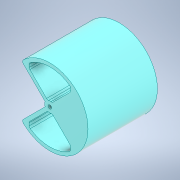
# Autodesk Inventor part: Feeder Rotator
Saved by Autodesk Inventor 2020.3 (Build 243373000, 373)
## iProperties
Created: 2020-07-23
Part Number: Feeder Rotator
Material: ABS Plastic
Document SubType Name: Modeling
Designer: juanp
Density: 1.06 g/cm^3
Appearance: Smooth - White
Author: juanp
Autodesk Inventor part; units mm, degrees
ref_plane "YZ Plane" through (0, 0, 0) normal (1, 0, 0) x (0, 1, 0)
ref_plane "XZ Plane" through (0, 0, 0) normal (0, 1, 0) x (-1, 0, 0)
ref_plane "XY Plane" through (0, 0, 0) normal (0, 0, 1) x (1, 0, 0)
sketch "Sketch2" plane through (0, 0, 0) normal (0, 0, 1) x (1, 0, 0)
  arc A0 (20.126, -22.2473) -> (-20.126, -22.2473) centre (0, 0) ccw construction
  arc A1 (-24.3711, -22.2497) -> (-24.3711, 22.2497) centre (0, 0) ccw
  line L0 (32.9543, 32.9543) -> (23.3345, 23.3345) construction
  line L1 (-32.8174, 32.8174) -> (-23.3345, 23.3345) construction
  line L2 (23.3345, 23.3345) -> (-23.3345, -23.3345) construction
  line L3 (23.3345, -23.3345) -> (30.6779, -35.5804) construction
  line L4 (-23.3345, -23.3345) -> (-31.805, -34.2596) construction
  line L5 (-23.3345, 23.3345) -> (23.3345, -23.3345) construction
  line L6 (0, -33) -> (0, 33) construction
  line L7 (32.9543, 0) -> (-32.9543, 0) construction
  circle A2 centre (0, 0) radius 1.5
  circle A3 centre (0, 0) radius 4.5
  line L8 (4.0607, -1.9393) -> (22.2473, -20.126) construction
  line L9 (1.9393, -4.0607) -> (17.8, -19.9213)
  arc A4 (0, -30) -> (17.8, -24.1487) centre (0, 0) ccw
  line L10 (-1.9393, -4.0607) -> (-17.8, -19.9213)
  line L11 (-4.0607, -1.9393) -> (-22.2473, -20.126) construction
  line L12 (23.3345, 23.3345) -> (-23.3345, -23.3345) construction
  arc A5 (-20.126, -22.2473) -> (-17.8, -24.1487) centre (0, 0) ccw construction
  line L13 (17.8, -24.1487) -> (17.8, -19.9213)
  line L14 (-17.8, -24.1487) -> (-17.8, -19.9213)
  line L15 (17.8, -22.035) -> (-17.8, -22.035) construction
  arc A6 (-17.8, -24.1487) -> (0, -30) centre (0, 0) ccw
  line L16 (-17.8, -19.9213) -> (-20.126, -22.2473) construction
  line L17 (17.8, -19.9213) -> (20.126, -22.2473) construction
  arc A7 (17.8, -24.1487) -> (20.126, -22.2473) centre (0, 0) ccw construction
  line L18 (17.8, 19.9213) -> (20.126, 22.2473) construction
  arc A8 (20.126, 22.2473) -> (17.8, 24.1487) centre (0, 0) ccw construction
  arc A9 (-17.8, 24.1487) -> (-20.126, 22.2473) centre (0, 0) ccw construction
  line L19 (-17.8, 19.9213) -> (-20.126, 22.2473) construction
  line L20 (-1.9393, 4.0607) -> (-17.8, 19.9213)
  line L21 (1.9393, 4.0607) -> (17.8, 19.9213)
  line L22 (17.8, 24.1487) -> (17.8, 19.9213)
  arc A10 (17.8, 24.1487) -> (0, 30) centre (0, 0) ccw
  arc A11 (0, 30) -> (-17.8, 24.1487) centre (0, 0) ccw
  line L23 (-17.8, 24.1487) -> (-17.8, 19.9213)
  line L24 (4.0607, 1.9393) -> (22.2473, 20.126) construction
  line L25 (-4.0607, 1.9393) -> (-22.2473, 20.126) construction
  line L26 (-4.0607, 1.9393) -> (-24.3711, 22.2497)
  line L27 (-4.0607, -1.9393) -> (-24.3711, -22.2497)
  arc A12 (-24.3711, 22.2497) -> (-24.3711, -22.2497) centre (0, 0) ccw construction
  point P0 (0, -22.035)
  dimension "d32" = 60
  dimension "d33" = 3
  dimension "d34" = 3
  dimension "d35" = 3
  dimension "d36" = 1.5
  dimension "d37" = 3
  dimension "d38" = 35.6
  dimension "d43" = 45
  constraints: 56 end point, 30 point on circle, 17 symmetric about line, 13 centre point, 9 parallel, 5 midpoint, 4 coincident, 4 point on line, 2 vertical, 1 horizontal, 6 other
  measures "d32" diameter of A0
  measures "d33" radial gap between concentric circles of A0 A1
  measures "d34" diameter of A2
  measures "d35" radial gap between concentric circles of A2 A3
  measures "d36" distance between parallel lines of L9 L5
  measures "d37" distance between parallel lines of L9 L8
  measures "d38" distance of L15.start L15.end
  measures "d43" angle of L7 L2
extrude "Extrusion2" add sketch "Sketch2" along normal blind 60 contours L27 A3 L10 L14 A6 A4 L13 L9 L21 L22 A10 A11 L23 L20 L26 A1 | A3
fillet "Fillet2" radius 2 14 edges at (-24.3711, 22.2497, 30) (-24.3711, -22.2497, 30) (-17.8, -24.1487, 30) (-17.8, -19.9213, 30) (-17.8, 24.1487, 30) (-17.8, 19.9213, 30) (17.8, -24.1487, 30) (17.8, -19.9213, 30) (17.8, 19.9213, 30) (17.8, 24.1487, 30) (-1.9393, 4.0607, 30) (1.9393, 4.0607, 30) (-1.9393, -4.0607, 30) (1.9393, -4.0607, 30)
body "Solid2"
